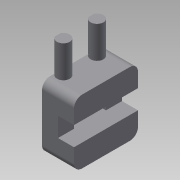
# Autodesk Inventor part: pig_torso
Saved by Autodesk Inventor 2015 (Build 190159000, 159)
## iProperties
Created: 2016-04-29
Part Number: pig_torso
Material: Generic
Document SubType Name: Modeling
Designer: Luke Good
Density: 1 g/cm^3
Appearance: Default
Author: Luke Good
Autodesk Inventor part; units mm, degrees
ref_plane "YZ Plane" through (0, 0, 0) normal (1, 0, 0) x (0, 1, 0)
ref_plane "XZ Plane" through (0, 0, 0) normal (0, 1, 0) x (-1, 0, 0)
ref_plane "XY Plane" through (0, 0, 0) normal (0, 0, 1) x (1, 0, 0)
sketch "Sketch1" plane through (0, 0, 0) normal (0, 0, 1) x (1, 0, 0)
  line L0 (6.35, -12.6955) -> (-6.35, -12.6955)
  line L1 (-6.35, -12.6955) -> (-6.35, 12.6955)
  line L2 (-6.35, 12.6955) -> (6.35, 12.6955)
  line L3 (6.35, 12.6955) -> (6.35, -12.6955)
  line L4 (6.35, -12.6955) -> (-6.35, 12.6955) construction
  line L5 (-6.35, -12.6955) -> (6.35, 12.6955) construction
  point P0 (0, 0)
  dimension "d1" = 0
  dimension "d0" = 12.7
  constraints: 12 end point, 4 point on line, 3 horizontal, 2 midpoint, 2 parallel, 2 vertical, 1 perpendicular, 8 other
  measures "d0" distance of L4.end L2.end
extrude "Extrusion1" add sketch "Sketch1" along normal blind 25.4
fillet "Fillet2" radius 3.175 4 edges at (0, 12.6955, 25.4) (0, -12.6955, 25.4) (0, 12.6955, 0) (0, -12.6955, 0)
sketch "Sketch4" plane through (6.35, -9.5205, 0) normal (1, 0, 0) x (0, 0, -1)
  line L0 (-25.4, 19.041) -> (-25.4, 0) projected
  line L1 (-25.4, 6.9805) -> (-25.4, 12.0605)
  line L2 (0, 12.0605) -> (0, 6.9805)
  line L3 (0, 6.9805) -> (-25.4, 12.0605) construction
  line L4 (-12.7, 9.5205) -> (0, 12.0605) construction
  line L5 (-9.3133, 6.9805) -> (-20.32, 15.2355) construction
  line L6 (-16.0867, 6.9805) -> (-5.08, 15.2355) construction
  line L7 (-4.2333, 6.9805) -> (-5.08, 6.9805)
  line L8 (-20.32, 6.9805) -> (-21.1667, 6.9805)
  line L9 (-25.4, 0) -> (-25.4, 19.041) projected
  line L10 (0, 5.7105) -> (-25.4, 5.7105)
  line L11 (-25.4, 5.7105) -> (-25.4, 13.3305)
  line L12 (-25.4, 13.3305) -> (0, 13.3305)
  line L13 (0, 13.3305) -> (0, 5.7105)
  line L14 (-25.4, 5.7105) -> (-21.1667, 6.9805) construction
  line L15 (-12.7, 9.5205) -> (0, 13.3305) construction
  line L16 (0, 5.7105) -> (-4.2333, 6.9805) construction
  line L17 (-12.7, 9.5205) -> (-25.4, 13.3305) construction
  point P0 (0, 9.5205)
  point P1 (-12.7, 9.5205)
  dimension "d32" = 7.62
  constraints: 32 end point, 6 point on line, 3 horizontal, 3 parallel, 3 perpendicular, 2 midpoint
  measures "d32" distance of L10.end L11.end
extrude "Extrusion4" cut sketch "Sketch4" against normal blind 6.35
sketch "Sketch6" plane through (-6.35, 12.6955, 3.175) normal (0, 1, 0) x (1, 0, 0)
  arc A0 (0, -3.7827) -> (0, -1.5483) centre (2.2811, -2.6655) ccw
  arc A1 (0, -17.1431) -> (0, -14.9087) centre (2.2811, -16.0259) ccw
  line L0 (0, 0) -> (0, -19.05) projected
  line L1 (0, -1.5483) -> (0, -3.7827)
  line L2 (0, -14.9087) -> (0, -17.1431)
  point P0 (6.35, 3.175)
  dimension "d22" = 5.08
  dimension "d24" = 5.08
  constraints: 4 end point, 4 point on circle, 4 point on line, 2 centre point, 2 collinear
  measures "d22" diameter of A0
  measures "d24" diameter of A1
extrude "Extrusion6" add sketch "Sketch6" along normal blind 12.7
sketch "Sketch7" plane through (0, -9.5205, 0) normal (1, 0, 0) x (0, 0, -1)
  line L0 (-6.35, 12.0605) -> (-6.35, 6.9805)
  line L1 (-19.05, 6.9805) -> (-19.05, 12.0605)
  line L2 (-19.05, 12.0605) -> (-6.35, 6.9805) construction
  line L3 (-6.35, 12.0605) -> (-19.05, 6.9805) construction
  line L4 (-6.35, 5.7105) -> (-19.05, 5.7105)
  line L5 (-19.05, 5.7105) -> (-19.05, 13.3305)
  line L6 (-19.05, 13.3305) -> (-6.35, 13.3305)
  line L7 (-6.35, 13.3305) -> (-6.35, 5.7105)
  line L8 (-6.35, 5.7105) -> (-19.05, 13.3305) construction
  line L9 (-19.05, 5.7105) -> (-6.35, 13.3305) construction
  point P0 (0, 9.5205)
  point P1 (-12.7, 9.5205)
  dimension "d29" = 12.7
  dimension "d33" = 12.7
  dimension "d34" = 7.62
  constraints: 20 end point, 4 midpoint, 3 parallel, 1 horizontal, 1 perpendicular
  measures "d29" distance of L0.end L1.start
  measures "d33" distance of L5.end L6.end
  measures "d34" distance of L4.end L5.end
extrude "Extrusion7" cut sketch "Sketch7" against normal blind 12.7
body "Solid1"
